Autodesk Fusion 360 part; units mm, degrees
(part 2 of 2)
sketch "Sketch7" plane through (-20, 0, 0) normal (-1, 0, 0) x (0, -1, 0) in component "ball"
  line L0 (15.0084, 21.0981) -> (-47.0084, 21.0981)
  line L1 (-45.8452, -1.5) -> (13.8452, -1.5)
  line L2 (-16, 21.0981) -> (-16, -1.5)
  spline S0 degree 5 poles (-16, 14) (-16.0768, 14.2889) (-16.2492, 14.8416) (-16.5647, 15.5947) (-17.0996, 16.4467) (-17.9572, 17.2552) (-18.9957, 17.8051) (-20.1949, 18.0972) (-21.5164, 18.1376) (-22.901, 17.9403) (-24.2811, 17.528) (-25.5916, 16.9332) (-26.7815, 16.2001) (-27.8246, 15.386) (-28.7338, 14.5642) (-29.5527, 13.8181) (-30.3405, 13.2309) (-31.1602, 12.878) (-32.064, 12.8165) (-33.0834, 13.0788) (-34.2362, 13.6807) (-35.2709, 14.4373) (-36.1107, 15.159) (-36.6989, 15.7083) (-37, 16) knots 0 0 0 0 0 0 0.05 0.1 0.15 0.2 0.25 0.3 0.35 0.4 0.45 0.5 0.55 0.6 0.65 0.7 0.75 0.8 0.85 0.9 0.95 1 1 1 1 1 1
  spline S1 degree 5 poles (-37, 16) (-37.054, 15.8762) (-37.1353, 15.6211) (-37.1776, 15.2158) (-37.0738, 14.6298) (-36.6785, 13.8269) (-36.0288, 12.9719) (-35.1528, 12.1033) (-34.1019, 11.2871) (-32.9409, 10.6016) (-31.738, 10.1239) (-30.5551, 9.9157) (-29.4385, 10.0096) (-28.4073, 10.3907) (-27.452, 10.9969) (-26.546, 11.7391) (-25.6526, 12.5164) (-24.7335, 13.2309) (-23.7575, 13.8057) (-22.7059, 14.1942) (-21.5684, 14.3708) (-20.5863, 14.3343) (-19.809, 14.2062) (-19.2727, 14.0762) (-19, 14) knots 0 0 0 0 0 0 0.05 0.1 0.15 0.2 0.25 0.3 0.35 0.4 0.45 0.5 0.55 0.6 0.65 0.7 0.75 0.8 0.85 0.9 0.95 1 1 1 1 1 1
  spline S2 degree 5 poles (-19, 14) (-19.1593, 13.9082) (-19.4654, 13.7188) (-19.8868, 13.4181) (-20.3668, 12.9863) (-20.8123, 12.4099) (-21.1083, 11.8121) (-21.3181, 11.2) (-21.5714, 10.5707) (-22.0076, 9.9217) (-22.7367, 9.2586) (-23.784, 8.6057) (-25.1061, 8.0019) (-26.6184, 7.4936) (-28.2175, 7.1291) (-29.8055, 6.952) (-31.3123, 6.9952) (-32.7222, 7.2735) (-34.063, 7.7868) (-35.3897, 8.5261) (-36.7709, 9.477) (-37.9734, 10.3947) (-38.9536, 11.1658) (-39.6449, 11.7159) (-40, 12) knots 0 0 0 0 0 0 0.05 0.1 0.15 0.2 0.25 0.3 0.35 0.4 0.45 0.5 0.55 0.6 0.65 0.7 0.75 0.8 0.85 0.9 0.95 1 1 1 1 1 1
  spline S3 degree 5 poles (-40, 12) (-39.9687, 11.8016) (-39.8965, 11.412) (-39.7599, 10.8497) (-39.5206, 10.1438) (-39.1227, 9.3355) (-38.6179, 8.6011) (-37.9915, 7.9389) (-37.2204, 7.3449) (-36.2794, 6.8136) (-35.1484, 6.3404) (-33.8195, 5.9223) (-32.3053, 5.5605) (-30.6447, 5.2605) (-28.8942, 5.0317) (-27.1214, 4.8852) (-25.3974, 4.8334) (-23.7904, 4.8877) (-22.359, 5.058) (-21.1435, 5.3502) (-20.1642, 5.7665) (-19.5763, 6.1986) (-19.2455, 6.5779) (-19.0737, 6.8552) (-19, 7) knots 0 0 0 0 0 0 0.05 0.1 0.15 0.2 0.25 0.3 0.35 0.4 0.45 0.5 0.55 0.6 0.65 0.7 0.75 0.8 0.85 0.9 0.95 1 1 1 1 1 1
  spline S4 degree 5 poles (-19, 7) (-19.0395, 6.762) (-19.1421, 6.3033) (-19.3671, 5.6668) (-19.795, 4.9205) (-20.4658, 4.1516) (-21.1809, 3.5372) (-21.8621, 3.0651) (-22.4694, 2.7196) (-23.0364, 2.481) (-23.646, 2.3283) (-24.3868, 2.2429) (-25.3204, 2.2114) (-26.4321, 2.2305) (-27.6344, 2.3056) (-28.8063, 2.4472) (-29.6176, 2.6233) (-30.1094, 2.7955) (-30.3795, 2.9288) (-30.5, 3) knots 0 0 0 0 0 0 0.066667 0.133333 0.2 0.266667 0.333333 0.4 0.466667 0.533333 0.6 0.666667 0.733333 0.8 0.866667 0.933333 1 1 1 1 1 1
  spline S5 degree 5 poles (-30.5, 3) (-30.428, 2.8413) (-30.2657, 2.5426) (-29.9676, 2.1509) (-29.4599, 1.7355) (-28.6407, 1.3622) (-27.6411, 1.096) (-26.4758, 0.9019) (-25.1766, 0.7599) (-23.7933, 0.6686) (-22.3845, 0.6374) (-21.0126, 0.6824) (-19.7366, 0.8207) (-18.6066, 1.0648) (-17.6554, 1.4167) (-16.8959, 1.8647) (-16.443, 2.287) (-16.1886, 2.633) (-16.0566, 2.8756) (-16, 3) knots 0 0 0 0 0 0 0.066667 0.133333 0.2 0.266667 0.333333 0.4 0.466667 0.533333 0.6 0.666667 0.733333 0.8 0.866667 0.933333 1 1 1 1 1 1
  spline S6 degree 5 poles (-16, 14) (-15.9232, 14.2889) (-15.7508, 14.8416) (-15.4353, 15.5947) (-14.9004, 16.4467) (-14.0428, 17.2552) (-13.0043, 17.8051) (-11.8051, 18.0972) (-10.4836, 18.1376) (-9.099, 17.9403) (-7.7189, 17.528) (-6.4084, 16.9332) (-5.2185, 16.2001) (-4.1754, 15.386) (-3.2662, 14.5642) (-2.4473, 13.8181) (-1.6595, 13.2309) (-0.8398, 12.878) (0.064, 12.8165) (1.0834, 13.0788) (2.2362, 13.6807) (3.2709, 14.4373) (4.1107, 15.159) (4.6989, 15.7083) (5, 16) knots 0 0 0 0 0 0 0.05 0.1 0.15 0.2 0.25 0.3 0.35 0.4 0.45 0.5 0.55 0.6 0.65 0.7 0.75 0.8 0.85 0.9 0.95 1 1 1 1 1 1
  line L3 (-15.2956, 11.3482) -> (-16.7044, 16.6518)
  line L4 (-34.3707, 13.4529) -> (-39.6293, 18.5471)
  line L5 (-16.7044, 11.3482) -> (-15.2956, 16.6518)
  line L6 (2.3707, 13.4529) -> (7.6293, 18.5471)
  spline S7 degree 5 poles (5, 16) (5.054, 15.8762) (5.1353, 15.6211) (5.1776, 15.2158) (5.0738, 14.6298) (4.6785, 13.8269) (4.0288, 12.9719) (3.1528, 12.1033) (2.1019, 11.2871) (0.9409, 10.6016) (-0.262, 10.1239) (-1.4449, 9.9157) (-2.5615, 10.0096) (-3.5927, 10.3907) (-4.548, 10.9969) (-5.454, 11.7391) (-6.3474, 12.5164) (-7.2665, 13.2309) (-8.2425, 13.8057) (-9.2941, 14.1942) (-10.4316, 14.3708) (-11.4137, 14.3343) (-12.191, 14.2062) (-12.7273, 14.0762) (-13, 14) knots 0 0 0 0 0 0 0.05 0.1 0.15 0.2 0.25 0.3 0.35 0.4 0.45 0.5 0.55 0.6 0.65 0.7 0.75 0.8 0.85 0.9 0.95 1 1 1 1 1 1
  line L7 (-36.4062, 17.3615) -> (-37.5938, 14.6385)
  line L8 (-21.2463, 14.6274) -> (-16.7537, 13.3726)
  line L9 (4.4062, 17.3615) -> (5.5938, 14.6385)
  line L10 (-10.7537, 14.6274) -> (-15.2463, 13.3726)
  spline S8 degree 5 poles (8, 12) (7.9687, 11.8016) (7.8965, 11.412) (7.7599, 10.8497) (7.5206, 10.1438) (7.1227, 9.3355) (6.6179, 8.6011) (5.9915, 7.9389) (5.2204, 7.3449) (4.2794, 6.8136) (3.1484, 6.3404) (1.8195, 5.9223) (0.3053, 5.5605) (-1.3553, 5.2605) (-3.1058, 5.0317) (-4.8786, 4.8852) (-6.6026, 4.8334) (-8.2096, 4.8877) (-9.641, 5.058) (-10.8565, 5.3502) (-11.8358, 5.7665) (-12.4237, 6.1986) (-12.7545, 6.5779) (-12.9263, 6.8552) (-13, 7) knots 0 0 0 0 0 0 0.05 0.1 0.15 0.2 0.25 0.3 0.35 0.4 0.45 0.5 0.55 0.6 0.65 0.7 0.75 0.8 0.85 0.9 0.95 1 1 1 1 1 1
  line L11 (-40.4106, 14.601) -> (-39.5894, 9.399)
  line L12 (-19.8094, 5.4101) -> (-18.1906, 8.5899)
  line L13 (8.4106, 14.601) -> (7.5894, 9.399)
  line L14 (-12.1906, 5.4101) -> (-13.8094, 8.5899)
  spline S9 degree 5 poles (-13, 7) (-12.9605, 6.762) (-12.8579, 6.3033) (-12.6329, 5.6668) (-12.205, 4.9205) (-11.5342, 4.1516) (-10.8191, 3.5372) (-10.1379, 3.0651) (-9.5306, 2.7196) (-8.9636, 2.481) (-8.354, 2.3283) (-7.6132, 2.2429) (-6.6796, 2.2114) (-5.5679, 2.2305) (-4.3656, 2.3056) (-3.1937, 2.4472) (-2.3824, 2.6233) (-1.8906, 2.7955) (-1.6205, 2.9288) (-1.5, 3) knots 0 0 0 0 0 0 0.066667 0.133333 0.2 0.266667 0.333333 0.4 0.466667 0.533333 0.6 0.666667 0.733333 0.8 0.866667 0.933333 1 1 1 1 1 1
  line L15 (-18.7185, 8.6976) -> (-19.2815, 5.3024)
  line L16 (-29.6914, 2.5221) -> (-31.3086, 3.4779)
  line L17 (-13.2815, 8.6976) -> (-12.7185, 5.3024)
  line L18 (-2.3086, 2.5221) -> (-0.6914, 3.4779)
  spline S10 degree 5 poles (-1.5, 3) (-1.572, 2.8413) (-1.7343, 2.5426) (-2.0324, 2.1509) (-2.5401, 1.7355) (-3.3593, 1.3622) (-4.3589, 1.096) (-5.5242, 0.9019) (-6.8234, 0.7599) (-8.2067, 0.6686) (-9.6155, 0.6374) (-10.9874, 0.6824) (-12.2634, 0.8207) (-13.3934, 1.0648) (-14.3446, 1.4167) (-15.1041, 1.8647) (-15.5571, 2.287) (-15.8114, 2.633) (-15.9434, 2.8756) (-16, 3) knots 0 0 0 0 0 0 0.066667 0.133333 0.2 0.266667 0.333333 0.4 0.466667 0.533333 0.6 0.666667 0.733333 0.8 0.866667 0.933333 1 1 1 1 1 1
  line L19 (-31.0931, 4.3075) -> (-29.9069, 1.6925)
  line L20 (-16.5066, 1.8872) -> (-15.4934, 4.1128)
  line L21 (-0.9069, 4.3075) -> (-2.0931, 1.6925)
  line L22 (-15.4934, 1.8872) -> (-16.5066, 4.1128)
  spline S11 degree 5 poles (-13, 14) (-12.8407, 13.9082) (-12.5346, 13.7188) (-12.1132, 13.4181) (-11.6332, 12.9863) (-11.1877, 12.4099) (-10.8917, 11.8121) (-10.6819, 11.2) (-10.4286, 10.5707) (-9.9924, 9.9217) (-9.2633, 9.2586) (-8.216, 8.6057) (-6.8939, 8.0019) (-5.3816, 7.4936) (-3.7825, 7.1291) (-2.1945, 6.952) (-0.6877, 6.9952) (0.7222, 7.2735) (2.063, 7.7868) (3.3897, 8.5261) (4.7709, 9.477) (5.9734, 10.3947) (6.9536, 11.1658) (7.6449, 11.7159) (8, 12) knots 0 0 0 0 0 0 0.05 0.1 0.15 0.2 0.25 0.3 0.35 0.4 0.45 0.5 0.55 0.6 0.65 0.7 0.75 0.8 0.85 0.9 0.95 1 1 1 1 1 1
  line L23 (-16.6348, 15.3636) -> (-21.3652, 12.6364)
  line L24 (-37.5, 10) -> (-42.5, 14)
  line L25 (-15.3652, 15.3636) -> (-10.6348, 12.6364)
  line L26 (5.5, 10) -> (10.5, 14)
  point P0 (-20, 18)
  point P1 (-27, 16)
  point P2 (-31, 13)
  point P3 (-36, 13)
  point P4 (-30, 10)
  point P5 (-25, 13)
  point P6 (-21, 12)
  point P7 (-22.1918, 9.799)
  point P8 (-30, 7)
  point P9 (-38.5308, 8.5504)
  point P10 (-34, 6)
  point P11 (-23, 5)
  point P12 (-22, 3)
  point P13 (-24.8082, 2.2362)
  point P14 (-27, 1)
  point P15 (-19, 1)
  point P16 (-12, 18)
  point P17 (-5, 16)
  point P18 (-1, 13)
  point P19 (4, 13)
  point P20 (-2, 10)
  point P21 (-7, 13)
  point P22 (6.5308, 8.5504)
  point P23 (2, 6)
  point P24 (-9, 5)
  point P25 (-10, 3)
  point P26 (-7.1918, 2.2362)
  point P27 (-5, 1)
  point P28 (-13, 1)
  point P29 (-11, 12)
  point P30 (-9.8082, 9.799)
  point P31 (-2, 7)
  constraint midpoint L0 L2.start
  constraint midpoint L1 L2.end
  constraint coincident L2 S0.start
  constraint coincident L2 S5.end
  constraint midpoint S0.start L3
  constraint midpoint S0.end L4
  constraint midpoint S0.end L7
  constraint midpoint S1.end L8
  constraint midpoint S2.end L11
  constraint midpoint S3.end L12
  constraint midpoint S3.end L15
  constraint midpoint S4.end L16
  constraint midpoint S4.end L19
  constraint midpoint S5.end L20
  constraint midpoint S1.end L23
  constraint midpoint S2.end L24
  constraint symmetric L2 S0.start S6.start
  constraint symmetric L2 P0 P16
  constraint symmetric L2 P1 P17
  constraint symmetric L2 P2 P18
  constraint symmetric L2 S0.end S6.end
  constraint symmetric L2 P3 P19
  constraint symmetric L2 P4 P20
  constraint symmetric L2 P5 P21
  constraint symmetric L2 S1.end S7.end
  constraint symmetric L2 P6 P29
  constraint symmetric L2 P7 P30
  constraint symmetric L2 P8 P31
  constraint symmetric L2 S2.end S8.start
  constraint symmetric L2 P9 P22
  constraint symmetric L2 P10 P23
  constraint symmetric L2 P11 P24
  constraint symmetric L2 S3.end S8.end
  constraint symmetric L2 P12 P25
  constraint symmetric L2 P13 P26
  constraint symmetric L2 S4.end S9.end
  constraint symmetric L2 P14 P27
  constraint symmetric L2 P15 P28
  constraint symmetric L2 S5.end S10.end
  constraint symmetric L2 L3.start L5.start
  constraint symmetric L2 L3.end L5.end
  constraint symmetric L2 L4.start L6.start
  constraint symmetric L2 L4.end L6.end
  constraint symmetric L2 L7.start L9.start
  constraint symmetric L2 L7.end L9.end
  constraint symmetric L2 L8.start L10.start
  constraint symmetric L2 L8.end L10.end
  constraint symmetric L2 L11.start L13.start
  constraint symmetric L2 L11.end L13.end
  constraint symmetric L2 L12.start L14.start
  constraint symmetric L2 L12.end L14.end
  constraint symmetric L2 L15.start L17.start
  constraint symmetric L2 L15.end L17.end
  constraint symmetric L2 L16.start L18.start
  constraint symmetric L2 L16.end L18.end
  constraint symmetric L2 L19.start L21.start
  constraint symmetric L2 L19.end L21.end
  constraint symmetric L2 L20.start L22.start
  constraint symmetric L2 L20.end L22.end
  constraint symmetric L2 L23.start L25.start
  constraint symmetric L2 L23.end L25.end
  constraint symmetric L2 L24.start L26.start
  constraint symmetric L2 L24.end L26.end
extrude "Extrude5'" cut sketch "Sketch7" against normal blind 25 bodies 2 in component "ball"
sketch "Sketch8" plane through (0, 0, 21.0981) normal (0, 0, 1) x (-1, 0, 0) in component "ball"
  circle A0 centre (-14.9383, -16) radius 31.0084
  circle A1 centre (-14.9383, -16) radius 29.4325
pattern_circular "C-Pattern1" count 3 over 360 about axis through (14.9566, 15.9909, -4.2) along (0, 0, 1) of "Extrude5'" in component "ball"
sketch "Sketch1 (4)" plane through (0, 0, -1.5) normal (0, 0, 1) x (-1, 0, 0) in component "extension"
  circle A0 centre (-42.0837, -16) radius 1
  circle A1 centre (12.2071, -16) radius 1
  circle A2 centre (-14.9383, -16) radius 29.8452
  arc A3 (13.1923, -13.9627) -> (-43.0689, -13.9627) centre (-14.9383, -16) ccw
  arc A4 (13.1923, -13.9627) -> (13.1923, -18.0373) centre (12.2071, -16) ccw
  arc A5 (-43.0689, -18.0373) -> (13.1923, -18.0373) centre (-14.9383, -16) ccw
  arc A6 (-43.0689, -18.0373) -> (-43.0689, -13.9627) centre (-42.0837, -16) ccw
  circle A7 centre (-14.9383, -16) radius 28.2043
  constraint concentric A2 A7
extrude "Extrude1'''" add sketch "Sketch1 (4)" along normal blind 10 separate body contours A2 makes body 6 in component "extension"
sketch "Sketch1 (5)" plane through (0, 16, 0) normal (0, 1, 0) x (1, 0, 0) in component "cap"
  spline S0 degree 3 poles (33.6875, -14) (34.5835, -14.3099) (35.3264, -14.3805) (36.6237, -14.1932) (37.1646, -13.937) (38.2798, -13.1441) (38.8055, -12.5318) (39.8448, -11.2941) (40.3568, -10.6687) (41.2779, -10.0864) (41.6509, -9.9614) (42.4833, -10.0177) (42.8832, -10.2011) (43.8376, -10.8937) (44.3591, -11.5742) (45.044, -12.8784) (45.2745, -13.5433) (45.4405, -14.5288) (45.458, -14.8297) (45.4481, -15.252) (45.4361, -15.408) (45.3915, -15.7167) (45.3607, -15.8616) (45.3214, -16) knots 0 0 0 0 0.347757 0.347757 0.693471 0.693471 1.163851 1.163851 1.680094 1.680094 1.993149 1.993149 2.311494 2.311494 2.845247 2.845247 3.301198 3.301198 3.550564 3.550564 3.691626 3.691626 3.827769 3.827769 3.827769 3.827769
  spline S1 degree 3 poles (45.3214, -16) (44.851, -14.667) (44.1735, -13.5705) (43.2036, -12.9208) (42.9372, -12.8567) (42.4624, -12.918) (42.2425, -13.0291) (41.7466, -13.4391) (41.4809, -13.7576) (40.4149, -15.1135) (39.2859, -16.6739) (36.5419, -17.9412) (35.6492, -18.1288) (34.2729, -18.0535) (33.7142, -17.9103) (32.7878, -17.3582) (32.4253, -17.0116) (31.8904, -16.2307) (31.7027, -15.8497) (31.3799, -14.9849) (31.2544, -14.4968) (31.1604, -14) knots 0 0 0 0 0.719439 0.719439 1.023307 1.023307 1.302416 1.302416 1.632983 1.632983 2.500728 2.500728 2.903769 2.903769 3.181925 3.181925 3.412664 3.412664 3.589293 3.589293 3.786428 3.786428 3.786428 3.786428
  spline S2 degree 3 poles (31.1604, -14) (30.9471, -14.7883) (30.625, -15.5542) (29.7972, -16.692) (29.3741, -17.0939) (28.3843, -17.7045) (27.849, -17.8961) (26.5454, -18.1356) (25.7656, -18.1111) (24.0487, -17.8187) (22.9402, -17.4516) (20.3642, -15.9895) (19.3561, -15.0245) (17.8649, -13.7598) (17.3075, -13.3425) (16.2925, -12.952) (15.8704, -12.8696) (14.94, -12.8938) (14.4385, -12.9877) (12.4362, -13.6838) (10.7904, -14.732) (8.9738, -16) knots 0 0 0 0 0.24545 0.24545 0.428593 0.428593 0.609942 0.609942 0.853396 0.853396 1.165598 1.165598 1.546937 1.546937 1.815146 1.815146 1.984101 1.984101 2.141432 2.141432 2.523706 2.523706 2.523706 2.523706
  spline S3 degree 3 poles (8.9738, -16) (8.9007, -15.8447) (8.8599, -15.682) (8.8432, -15.3308) (8.8718, -15.1525) (9.0066, -14.7139) (9.1484, -14.4577) (9.6196, -13.7713) (10.0734, -13.3075) (11.636, -11.9778) (13.104, -11.0415) (15.5333, -10.1392) (16.3608, -9.9836) (17.8575, -9.9873) (18.5032, -10.1416) (19.7788, -10.6838) (20.3858, -11.1044) (22.047, -12.4086) (23.0454, -13.384) (24.9981, -14.1786) (25.6423, -14.3085) (27.0539, -14.3401) (27.7918, -14.2124) (28.4941, -14) knots 0 0 0 0 0.051555 0.051555 0.106239 0.106239 0.191133 0.191133 0.360256 0.360256 0.704004 0.704004 0.918049 0.918049 1.127365 1.127365 1.370744 1.370744 1.820653 1.820653 2.036783 2.036783 2.278014 2.278014 2.278014 2.278014
  spline S4 degree 3 poles (28.4941, -14) (27.9198, -13.6274) (27.4521, -13.2065) (26.7871, -12.2856) (26.6289, -11.8776) (26.303, -10.9788) (26.134, -10.4635) (25.2167, -9.4348) (24.6854, -9.0762) (23.2362, -8.2376) (21.914, -7.7335) (19.1163, -7.0897) (17.2952, -6.8332) (13.104, -7.457) (11.3307, -8.4283) (8.376, -10.1195) (6.8875, -11.0228) (5.1481, -12) knots 0 0 0 0 0.223978 0.223978 0.425769 0.425769 0.683334 0.683334 0.903688 0.903688 1.384004 1.384004 1.830468 1.830468 2.346813 2.346813 2.720795 2.720795 2.720795 2.720795
  spline S5 degree 3 poles (5.1481, -12) (5.3651, -11.0862) (5.7294, -10.2289) (6.7885, -8.7676) (7.415, -8.205) (9.1019, -7.1287) (10.2386, -6.6768) (13.1879, -5.8121) (15.2978, -5.4029) (19.985, -4.8617) (22.0614, -4.7929) (24.8762, -5.0159) (25.9078, -5.2169) (27.0885, -5.7313) (27.4377, -5.9311) (28.0073, -6.4172) (28.2321, -6.6848) (28.3999, -7) knots 0 0 0 0 0.282973 0.282973 0.544611 0.544611 0.885334 0.885334 1.333576 1.333576 1.784582 1.784582 2.107176 2.107176 2.248199 2.248199 2.372209 2.372209 2.372209 2.372209
  spline S6 degree 3 poles (28.3999, -7) (28.2648, -6.3839) (28.0248, -5.7738) (27.2943, -4.6982) (26.8687, -4.2289) (25.9263, -3.4658) (25.5162, -3.1871) (24.3735, -2.5423) (23.792, -2.375) (22.1991, -2.1906) (20.9178, -2.2051) (19.0586, -2.3449) (18.3864, -2.419) (17.1043, -2.6679) (16.6547, -2.8222) (16.3428, -3) knots 0 0 0 0 0.189439 0.189439 0.338683 0.338683 0.43499 0.43499 0.611233 0.611233 0.834883 0.834883 0.9507 0.9507 1.077044 1.077044 1.077044 1.077044
  spline S7 degree 3 poles (16.3428, -3) (16.4515, -2.6984) (16.6108, -2.4295) (17.051, -1.962) (17.314, -1.7812) (17.9805, -1.4415) (18.4759, -1.2706) (20.4608, -0.8487) (22.4394, -0.6505) (25.8671, -0.6605) (27.3044, -0.8009) (28.9519, -1.4217) (29.4224, -1.6667) (30.0045, -2.1413) (30.1671, -2.2991) (30.4481, -2.6365) (30.5672, -2.8119) (30.6663, -3) knots 0 0 0 0 0.099523 0.099523 0.198309 0.198309 0.329298 0.329298 0.572591 0.572591 0.764033 0.764033 0.842721 0.842721 0.87626 0.87626 0.907407 0.907407 0.907407 0.907407
  spline S8 degree 3 poles (30.6663, -3) (30.7458, -2.6956) (30.8801, -2.4264) (31.2887, -1.8693) (31.5915, -1.6184) (32.4808, -1.0857) (33.1408, -0.9004) (35.0678, -0.5764) (36.6328, -0.6289) (38.7398, -0.9438) (39.5092, -1.12) (40.3992, -1.6121) (40.6501, -1.8101) (40.9801, -2.1866) (41.0833, -2.3273) (41.2776, -2.6453) (41.3647, -2.8178) (41.4421, -3) knots 0 0 0 0 0.103254 0.103254 0.245243 0.245243 0.492345 0.492345 1.006021 1.006021 1.302991 1.302991 1.4497 1.4497 1.524204 1.524204 1.600684 1.600684 1.600684 1.600684
  spline S9 degree 3 poles (41.4421, -3) (41.3064, -2.8844) (41.122, -2.7638) (40.3496, -2.4439) (39.668, -2.3157) (38.2978, -2.2122) (37.714, -2.2111) (36.6305, -2.3246) (36.2201, -2.4828) (35.558, -2.9993) (35.3403, -3.2054) (34.8188, -3.767) (34.4502, -4.2363) (34.0035, -5.1404) (33.8784, -5.4666) (33.6827, -6.1967) (33.6212, -6.5886) (33.5933, -7) knots 0 0 0 0 0.071077 0.071077 0.202116 0.202116 0.301066 0.301066 0.433215 0.433215 0.497193 0.497193 0.601672 0.601672 0.654922 0.654922 0.712197 0.712197 0.712197 0.712197
  spline S10 degree 3 poles (33.5933, -7) (33.6954, -6.7073) (33.8422, -6.4553) (34.2623, -5.9493) (34.5538, -5.731) (35.3777, -5.2712) (36.012, -5.0863) (37.9573, -4.7815) (39.5189, -4.829) (42.9628, -5.4691) (44.2979, -6.0911) (45.6177, -7.4892) (45.9305, -8.0788) (46.3114, -9.1921) (46.4296, -9.6814) (46.6082, -10.7829) (46.663, -11.3805) (46.685, -12) knots 0 0 0 0 0.099847 0.099847 0.232599 0.232599 0.463962 0.463962 0.892506 0.892506 1.441385 1.441385 1.761402 1.761402 1.968837 1.968837 2.183845 2.183845 2.183845 2.183845
  spline S11 degree 3 poles (46.685, -12) (46.1256, -10.5333) (45.2652, -9.1251) (43.7522, -7.5542) (43.0251, -7.1088) (41.1603, -6.9206) (40.1694, -7.2049) (38.4215, -7.9487) (37.5261, -8.4981) (36.3683, -9.5833) (36.0941, -10.005) (35.7431, -10.7177) (35.6431, -11.0736) (35.4034, -11.8712) (35.2559, -12.3177) (34.6195, -13.2447) (34.2072, -13.6444) (33.6875, -14) knots 0 0 0 0 0.936383 0.936383 1.666398 1.666398 2.412456 2.412456 3.226486 3.226486 3.826518 3.826518 4.477931 4.477931 5.331592 5.331592 6.127336 6.127336 6.127336 6.127336
  spline S12 degree 3 poles (28.4691, -14) (27.4442, -14.3098) (26.5497, -14.3804) (24.9605, -14.1933) (24.2802, -13.9372) (22.8431, -13.1447) (22.1327, -12.5327) (20.6229, -11.295) (19.815, -10.6691) (18.2636, -10.0866) (17.6166, -9.9616) (16.1106, -10.0174) (15.3545, -10.2005) (13.448, -10.8916) (12.2738, -11.5708) (10.4887, -12.8745) (9.7576, -13.5402) (9.091, -14.481) (8.9297, -14.7907) (8.8209, -15.2514) (8.8058, -15.4075) (8.8332, -15.7165) (8.873, -15.8614) (8.9382, -16) knots 0 0 0 0 0.347643 0.347643 0.693187 0.693187 1.163217 1.163217 1.679374 1.679374 1.992094 1.992094 2.310026 2.310026 2.842782 2.842782 3.298879 3.298879 3.515565 3.515565 3.623015 3.623015 3.726706 3.726706 3.726706 3.726706
  spline S13 degree 3 poles (8.9382, -16) (10.8501, -14.6665) (12.5794, -13.5699) (14.6815, -12.9207) (15.2141, -12.8567) (16.1229, -12.9181) (16.5239, -13.029) (17.3846, -13.4386) (17.8183, -13.7569) (19.4579, -15.1132) (21.0099, -16.6762) (24.4412, -17.9422) (25.5218, -18.1291) (27.1818, -18.053) (27.8542, -17.9095) (28.991, -17.357) (29.4454, -17.0103) (30.1357, -16.2292) (30.3855, -15.8485) (30.8247, -14.9841) (31.0023, -14.4964) (31.1366, -14) knots 0 0 0 0 0.7191 0.7191 1.022584 1.022584 1.301348 1.301348 1.631598 1.631598 2.499929 2.499929 2.902346 2.902346 3.180099 3.180099 3.410615 3.410615 3.586985 3.586985 3.783824 3.783824 3.783824 3.783824
  spline S14 degree 3 poles (31.1366, -14) (31.2859, -14.7883) (31.5143, -15.5542) (32.1445, -16.692) (32.4767, -17.094) (33.2759, -17.7046) (33.7172, -17.8961) (34.7972, -18.1356) (35.4463, -18.1111) (36.8558, -17.8185) (37.7534, -17.4512) (39.7475, -15.9882) (40.4738, -15.0229) (41.4595, -13.7588) (41.7987, -13.342) (42.3709, -12.9517) (42.5988, -12.8694) (43.074, -12.894) (43.3197, -12.9882) (44.2274, -13.6852) (44.861, -14.733) (45.3094, -16) knots 0 0 0 0 0.245461 0.245461 0.428639 0.428639 0.610036 0.610036 0.853579 0.853579 1.165847 1.165847 1.54722 1.54722 1.81505 1.81505 1.98398 1.98398 2.141333 2.141333 2.523101 2.523101 2.523101 2.523101
  spline S15 degree 3 poles (45.3094, -16) (45.3536, -15.8449) (45.3868, -15.6824) (45.4322, -15.3316) (45.4416, -15.1536) (45.4399, -14.7156) (45.4144, -14.4599) (45.3052, -13.7749) (45.1711, -13.3121) (44.6299, -11.9842) (44.0115, -11.0485) (42.8001, -10.1422) (42.3529, -9.9849) (41.5215, -9.986) (41.1498, -10.1363) (40.39, -10.6677) (40.0101, -11.0824) (38.9004, -12.3849) (38.1557, -13.3696) (36.6049, -14.1746) (36.0818, -14.307) (34.9102, -14.3412) (34.2823, -14.2134) (33.665, -14) knots 0 0 0 0 0.051503 0.051503 0.106111 0.106111 0.190848 0.190848 0.359591 0.359591 0.702822 0.702822 0.917286 0.917286 1.124895 1.124895 1.367315 1.367315 1.820839 1.820839 2.038753 2.038753 2.281958 2.281958 2.281958 2.281958
  spline S16 degree 3 poles (33.665, -14) (34.2099, -13.6274) (34.6391, -13.2065) (35.2399, -12.2856) (35.3786, -11.8775) (35.6517, -10.9788) (35.7848, -10.4635) (36.4778, -9.435) (36.8694, -9.0764) (37.9089, -8.2379) (38.8123, -7.734) (40.5613, -7.0899) (41.6275, -6.8331) (43.8442, -7.4589) (44.6739, -8.4373) (45.8085, -10.1242) (46.3028, -11.0253) (46.6763, -12) knots 0 0 0 0 0.223989 0.223989 0.425782 0.425782 0.683335 0.683335 0.903686 0.903686 1.383974 1.383974 1.830669 1.830669 2.349416 2.349416 2.72575 2.72575 2.72575 2.72575
  spline S17 degree 3 poles (46.6763, -12) (46.6436, -11.0864) (46.5403, -10.2295) (46.1893, -8.7685) (45.9675, -8.206) (45.3332, -7.1299) (44.8807, -6.6777) (43.5649, -5.8135) (42.5248, -5.405) (39.7485, -4.8619) (38.3066, -4.7925) (36.241, -5.0162) (35.4436, -5.2172) (34.5355, -5.7315) (34.2675, -5.9313) (33.8425, -6.4173) (33.6808, -6.6849) (33.5708, -7) knots 0 0 0 0 0.282943 0.282943 0.544668 0.544668 0.885418 0.885418 1.332124 1.332124 1.784181 1.784181 2.106506 2.106506 2.247435 2.247435 2.371367 2.371367 2.371367 2.371367
  spline S18 degree 3 poles (33.5708, -7) (33.6126, -6.384) (33.7327, -5.774) (34.1741, -4.6993) (34.4466, -4.2299) (35.0618, -3.4661) (35.3303, -3.1874) (36.0823, -2.5422) (36.4807, -2.3749) (37.6015, -2.1906) (38.4962, -2.2051) (39.7085, -2.3449) (40.1335, -2.419) (40.9359, -2.6679) (41.2167, -2.8223) (41.4255, -3) knots 0 0 0 0 0.189406 0.189406 0.338408 0.338408 0.434439 0.434439 0.610281 0.610281 0.833323 0.833323 0.948795 0.948795 1.074788 1.074788 1.074788 1.074788
  spline S19 degree 3 poles (41.4255, -3) (41.2974, -2.6985) (41.1453, -2.4297) (40.7832, -1.9624) (40.5875, -1.7815) (40.1125, -1.4418) (39.7759, -1.271) (38.4231, -0.8484) (37.0319, -0.6498) (34.3644, -0.661) (33.1718, -0.8018) (31.8512, -1.4228) (31.4814, -1.6677) (31.0575, -2.1419) (30.944, -2.2997) (30.7619, -2.6368) (30.6917, -2.812) (30.6426, -3) knots 0 0 0 0 0.099483 0.099483 0.198242 0.198242 0.329249 0.329249 0.573183 0.573183 0.76449 0.76449 0.843109 0.843109 0.876624 0.876624 0.907752 0.907752 0.907752 0.907752
  spline S20 degree 3 poles (30.6426, -3) (30.4821, -2.6956) (30.2704, -2.4265) (29.6871, -1.8695) (29.292, -1.6186) (28.1656, -1.0859) (27.3631, -0.9007) (24.9865, -0.5765) (22.9838, -0.6287) (20.0091, -0.9433) (18.8546, -1.1195) (17.5672, -1.6116) (17.2177, -1.8097) (16.7988, -2.1863) (16.6757, -2.327) (16.4627, -2.6451) (16.3776, -2.8177) (16.3119, -3) knots 0 0 0 0 0.103229 0.103229 0.245156 0.245156 0.492116 0.492116 1.005373 1.005373 1.302444 1.302444 1.44921 1.44921 1.523743 1.523743 1.600256 1.600256 1.600256 1.600256
  spline S21 degree 3 poles (16.3119, -3) (16.515, -2.8843) (16.8039, -2.7637) (18.0377, -2.4439) (19.1347, -2.3158) (21.1989, -2.2122) (22.0385, -2.211) (23.5808, -2.3246) (24.1717, -2.4827) (25.1746, -2.9988) (25.5076, -3.205) (26.305, -3.7664) (26.8674, -4.2358) (27.5849, -5.1401) (27.7944, -5.4664) (28.151, -6.1966) (28.2846, -6.5885) (28.3749, -7) knots 0 0 0 0 0.071123 0.071123 0.202326 0.202326 0.301499 0.301499 0.433869 0.433869 0.498001 0.498001 0.602731 0.602731 0.656106 0.656106 0.71352 0.71352 0.71352 0.71352
  spline S22 degree 3 poles (28.3749, -7) (28.219, -6.7073) (28.0137, -6.4553) (27.4478, -5.9493) (27.0679, -5.7311) (25.9963, -5.2713) (25.1744, -5.0863) (22.5568, -4.7815) (20.343, -4.829) (14.4889, -5.4781) (11.4767, -6.121) (8.2709, -7.558) (7.4251, -8.1404) (6.3587, -9.269) (6.0194, -9.748) (5.4593, -10.8197) (5.2521, -11.3997) (5.1094, -12) knots 0 0 0 0 0.09984 0.09984 0.232561 0.232561 0.463842 0.463842 0.892231 0.892231 1.454718 1.454718 1.754316 1.754316 1.939512 1.939512 2.131773 2.131773 2.131773 2.131773
  spline S23 degree 3 poles (5.1094, -12) (7.7236, -10.5327) (9.9081, -9.1247) (13.2407, -7.5544) (14.6823, -7.1092) (18.1051, -6.9204) (19.7639, -7.2043) (22.4998, -7.9471) (23.7819, -8.497) (25.3697, -9.5829) (25.7271, -10.0047) (26.1852, -10.7174) (26.3117, -11.0734) (26.6002, -11.8713) (26.7683, -12.3177) (27.4718, -13.2447) (27.9208, -13.6444) (28.4691, -14) knots 0 0 0 0 0.935585 0.935585 1.664592 1.664592 2.409964 2.409964 3.225511 3.225511 3.826201 3.826201 4.478452 4.478452 5.333957 5.333957 6.13181 6.13181 6.13181 6.13181
  spline S24 degree 3 poles (-17.3155, -14) (-17.187, -14.3098) (-17.0357, -14.3804) (-16.7444, -14.1933) (-16.6053, -13.9372) (-16.2838, -13.1447) (-16.0993, -12.5326) (-15.6296, -11.295) (-15.3343, -10.6691) (-14.7049, -10.0866) (-14.431, -9.9616) (-13.7577, -10.0174) (-13.4016, -10.2005) (-12.4498, -10.8918) (-11.7974, -11.5711) (-10.6993, -12.8748) (-10.2001, -13.5404) (-9.6928, -14.4811) (-9.558, -14.7908) (-9.4386, -15.2514) (-9.4116, -15.4075) (-9.3944, -15.7165) (-9.4034, -15.8615) (-9.4291, -16) knots 0 0 0 0 0.347651 0.347651 0.693206 0.693206 1.16326 1.16326 1.679422 1.679422 1.992164 1.992164 2.310124 2.310124 2.842947 2.842947 3.299034 3.299034 3.515711 3.515711 3.623164 3.623164 3.726858 3.726858 3.726858 3.726858
  spline S25 degree 3 poles (-9.4291, -16) (-10.869, -14.6666) (-11.9194, -13.5699) (-13.0504, -12.9207) (-13.3166, -12.8567) (-13.7504, -12.9181) (-13.9314, -13.029) (-14.2959, -13.4386) (-14.4639, -13.7569) (-15.0361, -15.1132) (-15.4567, -16.676) (-16.14, -17.9421) (-16.328, -18.1291) (-16.6117, -18.053) (-16.7255, -17.9095) (-16.936, -17.3571) (-17.0279, -17.0104) (-17.1834, -16.2293) (-17.2456, -15.8486) (-17.3623, -14.9842) (-17.4144, -14.4964) (-17.4547, -14) knots 0 0 0 0 0.719123 0.719123 1.022632 1.022632 1.30142 1.30142 1.63169 1.63169 2.499983 2.499983 2.902442 2.902442 3.180221 3.180221 3.410752 3.410752 3.587139 3.587139 3.783998 3.783998 3.783998 3.783998
  spline S26 degree 3 poles (-17.4547, -14) (-17.3906, -14.7883) (-17.2967, -15.5542) (-17.0988, -16.692) (-17.0077, -17.094) (-16.8166, -17.7045) (-16.7222, -17.8961) (-16.4978, -18.1356) (-16.3665, -18.1111) (-16.0581, -17.8185) (-15.8464, -17.4513) (-15.2626, -15.9883) (-14.9802, -15.023) (-14.4744, -13.7589) (-14.2562, -13.3421) (-13.8132, -12.9518) (-13.6185, -12.8694) (-13.162, -12.8939) (-12.9056, -12.9881) (-11.8098, -13.6851) (-10.7973, -14.7329) (-9.4291, -16) knots 0 0 0 0 0.245461 0.245461 0.428636 0.428636 0.61003 0.61003 0.853567 0.853567 1.16583 1.16583 1.547201 1.547201 1.815056 1.815056 1.983988 1.983988 2.14134 2.14134 2.523141 2.523141 2.523141 2.523141
  spline S27 degree 3 poles (-9.4291, -16) (-9.4003, -15.8449) (-9.3926, -15.6823) (-9.4212, -15.3316) (-9.4591, -15.1535) (-9.5917, -14.7155) (-9.7076, -14.4597) (-10.0684, -13.7746) (-10.3868, -13.3118) (-11.405, -11.9838) (-12.2527, -11.048) (-13.4718, -10.142) (-13.8542, -9.9848) (-14.5152, -9.9861) (-14.7842, -10.1365) (-15.2928, -10.668) (-15.5178, -11.0828) (-16.0759, -12.3854) (-16.3326, -13.3698) (-16.742, -14.1747) (-16.8659, -14.3071) (-17.1131, -14.3412) (-17.227, -14.2134) (-17.3155, -14) knots 0 0 0 0 0.051507 0.051507 0.106119 0.106119 0.190867 0.190867 0.359636 0.359636 0.702902 0.702902 0.917338 0.917338 1.124926 1.124926 1.367342 1.367342 1.820765 1.820765 2.038629 2.038629 2.281779 2.281779 2.281779 2.281779
  spline S28 degree 3 poles (-17.3155, -14) (-17.2858, -13.6274) (-17.2471, -13.2065) (-17.1826, -12.2856) (-17.163, -11.8775) (-17.11, -10.9788) (-17.0741, -10.4635) (-16.8496, -9.435) (-16.7097, -9.0764) (-16.2998, -8.2379) (-15.881, -7.734) (-14.831, -7.0899) (-14.0742, -6.8331) (-12.0859, -7.4588) (-11.1362, -8.437) (-9.3227, -10.1238) (-8.3305, -11.0251) (-6.9671, -12) knots 0 0 0 0 0.223989 0.223989 0.425782 0.425782 0.683336 0.683336 0.903689 0.903689 1.38398 1.38398 1.830653 1.830653 2.3493 2.3493 2.725624 2.725624 2.725624 2.725624
  spline S29 degree 3 poles (-6.9671, -12) (-7.1516, -11.0864) (-7.4127, -10.2294) (-8.1212, -8.7685) (-8.5262, -8.2059) (-9.5789, -7.1298) (-10.2636, -6.6776) (-11.8965, -5.8134) (-12.9619, -5.4049) (-14.8772, -4.8619) (-15.5194, -4.7926) (-16.2735, -5.0162) (-16.5076, -5.2172) (-16.7802, -5.7315) (-16.8614, -5.9313) (-17.0061, -6.4173) (-17.0693, -6.6848) (-17.1272, -7) knots 0 0 0 0 0.282945 0.282945 0.544664 0.544664 0.885464 0.885464 1.332424 1.332424 1.784563 1.784563 2.107015 2.107015 2.247997 2.247997 2.371977 2.371977 2.371977 2.371977
  spline S30 degree 3 poles (-17.1272, -7) (-17.0337, -6.384) (-16.9139, -5.774) (-16.6249, -4.6984) (-16.472, -4.2292) (-16.1439, -3.4661) (-16.0022, -3.1873) (-15.6105, -2.5423) (-15.4269, -2.3749) (-14.954, -2.1906) (-14.5668, -2.2051) (-13.9189, -2.3449) (-13.6715, -2.419) (-13.1911, -2.6679) (-13.022, -2.8223) (-12.9189, -3) knots 0 0 0 0 0.189408 0.189408 0.33867 0.33867 0.435011 0.435011 0.611411 0.611411 0.835168 0.835168 0.951012 0.951012 1.07741 1.07741 1.07741 1.07741
  spline S31 degree 3 poles (-12.9189, -3) (-12.8995, -2.6985) (-12.9067, -2.4297) (-12.9848, -1.9624) (-13.0521, -1.7815) (-13.2436, -1.4418) (-13.4025, -1.271) (-14.037, -0.8484) (-14.6302, -0.6499) (-15.393, -0.661) (-15.6365, -0.8017) (-15.9622, -1.4227) (-16.0625, -1.6677) (-16.2201, -2.1419) (-16.2691, -2.2997) (-16.3678, -2.6368) (-16.4166, -2.812) (-16.4667, -3) knots 0 0 0 0 0.099485 0.099485 0.198246 0.198246 0.329252 0.329252 0.573143 0.573143 0.764459 0.764459 0.843083 0.843083 0.8766 0.8766 0.907729 0.907729 0.907729 0.907729
  spline S32 degree 3 poles (-16.4667, -3) (-16.3856, -2.6956) (-16.3083, -2.4265) (-16.1338, -1.8695) (-16.0415, -1.6186) (-15.8046, -1.0859) (-15.6621, -0.9007) (-15.2126, -0.5765) (-14.7749, -0.6288) (-13.9096, -0.9433) (-13.5258, -1.1195) (-13.1299, -1.6116) (-13.0317, -1.8097) (-12.9432, -2.1863) (-12.9235, -2.3271) (-12.905, -2.6451) (-12.9072, -2.8177) (-12.9189, -3) knots 0 0 0 0 0.10323 0.10323 0.245162 0.245162 0.492131 0.492131 1.005416 1.005416 1.30248 1.30248 1.449243 1.449243 1.523774 1.523774 1.600285 1.600285 1.600285 1.600285
  spline S33 degree 3 poles (-12.9189, -3) (-12.986, -2.8843) (-13.0903, -2.7637) (-13.5514, -2.4439) (-13.9664, -2.3158) (-14.6596, -2.2122) (-14.9147, -2.211) (-15.3725, -2.3246) (-15.5529, -2.4827) (-15.8934, -2.9989) (-16.0085, -3.205) (-16.2841, -3.7665) (-16.4775, -4.2358) (-16.7478, -5.1402) (-16.8321, -5.4664) (-16.9928, -6.1966) (-17.0648, -6.5885) (-17.1272, -7) knots 0 0 0 0 0.07112 0.07112 0.202312 0.202312 0.301471 0.301471 0.433826 0.433826 0.497948 0.497948 0.602659 0.602659 0.656026 0.656026 0.713429 0.713429 0.713429 0.713429
  spline S34 degree 3 poles (-17.1272, -7) (-17.0734, -6.7073) (-17.015, -6.4553) (-16.8695, -5.9493) (-16.7812, -5.7311) (-16.5339, -5.2713) (-16.3466, -5.0863) (-15.6754, -4.7815) (-15.0242, -4.829) (-12.6662, -5.4781) (-11.0163, -6.1209) (-9.0961, -7.5578) (-8.5567, -8.1402) (-7.8614, -9.2689) (-7.634, -9.7479) (-7.2433, -10.8197) (-7.0884, -11.3997) (-6.9671, -12) knots 0 0 0 0 0.09984 0.09984 0.232564 0.232564 0.46385 0.46385 0.892249 0.892249 1.454723 1.454723 1.754409 1.754409 1.939671 1.939671 2.131999 2.131999 2.131999 2.131999
  spline S35 degree 3 poles (-6.9671, -12) (-9.019, -10.5328) (-10.3418, -9.1247) (-12.1595, -7.5544) (-12.8737, -7.1091) (-14.4311, -6.9204) (-15.0989, -7.2043) (-16.0858, -7.9472) (-16.4705, -8.4971) (-16.8987, -9.583) (-16.9817, -10.0047) (-17.0885, -10.7175) (-17.1149, -11.0735) (-17.1635, -11.8713) (-17.184, -12.3177) (-17.2507, -13.2447) (-17.2872, -13.6444) (-17.3155, -14) knots 0 0 0 0 0.935639 0.935639 1.664713 1.664713 2.410131 2.410131 3.225575 3.225575 3.826221 3.826221 4.478416 4.478416 5.333797 5.333797 6.131509 6.131509 6.131509 6.131509
  line L0 (-16.0701, -21.0981) -> (45.9467, -21.0981)
  line L1 (44.7834, 1.5) -> (-14.9069, 1.5)
  line L2 (14.9383, -21.0981) -> (14.9383, -44)
  circle A0 centre (14.9383, -11.3653) radius 32.5
  circle A1 centre (14.9383, -11.3653) radius 31
  line L3 (-16.0701, -21.0981) -> (45.9467, -21.0981)
  constraint midpoint L0 L2.start
  constraint perpendicular L0 L2
revolve "Revolve1'" add sketch "Sketch1 (5)" angle 360 about axis through (14.9383, 16, 21.0981) along (0, 0, 1) separate body contours L0 L2 A0 A1 L3 picked at (43.7945, -23.8444) makes body 7 in component "cap"
sketch "Sketch2 (4)" plane through (-20, 0, 0) normal (-1, 0, 0) x (0, -1, 0) in component "cap"
  spline S0 degree 5 poles (-3, 22) (-3.0117, 22.0801) (-3.0541, 22.2598) (-3.1749, 22.5874) (-3.4504, 23.1408) (-3.986, 24.0149) (-4.7142, 25.0354) (-5.6368, 26.1301) (-6.753, 27.2066) (-8.0574, 28.1655) (-9.5362, 28.9152) (-11.1651, 29.3858) (-12.9055, 29.545) (-14.7088, 29.3971) (-16.5238, 28.9744) (-18.3035, 28.3312) (-20.0119, 27.5371) (-21.6305, 26.6707) (-23.1666, 25.8125) (-24.6535, 25.0397) (-26.134, 24.423) (-27.6494, 24.0232) (-29.2242, 23.8874) (-30.8554, 24.0463) (-32.495, 24.509) (-34.0529, 25.2637) (-35.4173, 26.2801) (-36.47, 27.512) (-37.1039, 28.8997) (-37.2395, 30.3725) (-36.8421, 31.8509) (-35.9204, 33.2509) (-34.5225, 34.4897) (-32.7336, 35.4891) (-30.6732, 36.1815) (-28.4929, 36.5138) (-26.3716, 36.4524) (-24.4933, 35.9887) (-23.028, 35.1439) (-22.1099, 33.9745) (-21.8193, 32.5768) (-22.1576, 31.0956) (-23.0398, 29.7174) (-24.3244, 28.631) (-25.8357, 27.9929) (-27.3885, 27.8932) (-28.8131, 28.3146) (-29.9747, 29.115) (-30.7684, 30.0886) (-31.1183, 31.0141) (-30.9752, 31.7075) (-30.4471, 32.0021) (-29.8152, 32.0632) (-29.2892, 32.0329) (-29, 32) knots 0 0 0 0 0 0 0.02 0.04 0.06 0.08 0.1 0.12 0.14 0.16 0.18 0.2 0.22 0.24 0.26 0.28 0.3 0.32 0.34 0.36 0.38 0.4 0.42 0.44 0.46 0.48 0.5 0.52 0.54 0.56 0.58 0.6 0.62 0.64 0.66 0.68 0.7 0.72 0.74 0.76 0.78 0.8 0.82 0.84 0.86 0.88 0.9 0.92 0.94 0.96 0.98 1 1 1 1 1 1
  spline S1 degree 5 poles (-29, 32) (-29.0202, 31.8673) (-29.0241, 31.6237) (-28.9201, 31.3235) (-28.5626, 31.0541) (-27.7872, 30.932) (-26.8047, 31.0144) (-25.8314, 31.2808) (-25.0998, 31.7006) (-24.8045, 32.2332) (-25.0226, 32.8264) (-25.7015, 33.4185) (-26.72, 33.9432) (-27.9297, 34.3332) (-29.2095, 34.5246) (-30.4678, 34.4637) (-31.6323, 34.1146) (-32.6445, 33.4682) (-33.4525, 32.5476) (-34.0027, 31.4203) (-34.2416, 30.1915) (-34.1265, 28.9823) (-33.6356, 27.9119) (-32.7758, 27.0799) (-31.596, 26.5435) (-30.1831, 26.3148) (-28.6432, 26.3733) (-27.0879, 26.6749) (-25.6175, 27.1617) (-24.3069, 27.7718) (-23.1868, 28.4495) (-22.2393, 29.1517) (-21.4158, 29.8448) (-20.6507, 30.505) (-19.8759, 31.1164) (-19.0355, 31.6708) (-18.0987, 32.1657) (-17.0535, 32.6015) (-15.9041, 32.9783) (-14.6667, 33.2928) (-13.3661, 33.5348) (-12.0318, 33.6847) (-10.6964, 33.7161) (-9.3931, 33.599) (-8.1544, 33.3023) (-7.0094, 32.7966) (-5.9823, 32.0575) (-5.0907, 31.0676) (-4.3467, 29.8147) (-3.7582, 28.2914) (-3.3298, 26.4935) (-3.1167, 24.8342) (-3.0299, 23.4655) (-3.0046, 22.4977) (-3, 22) knots 0 0 0 0 0 0 0.02 0.04 0.06 0.08 0.1 0.12 0.14 0.16 0.18 0.2 0.22 0.24 0.26 0.28 0.3 0.32 0.34 0.36 0.38 0.4 0.42 0.44 0.46 0.48 0.5 0.52 0.54 0.56 0.58 0.6 0.62 0.64 0.66 0.68 0.7 0.72 0.74 0.76 0.78 0.8 0.82 0.84 0.86 0.88 0.9 0.92 0.94 0.96 0.98 1 1 1 1 1 1
  spline S2 degree 5 poles (-20.2205, 38.2828) (-20.2657, 38.4037) (-20.3393, 38.6376) (-20.3992, 38.965) (-20.3778, 39.3547) (-20.1823, 39.762) (-19.8233, 40.0873) (-19.3141, 40.3273) (-18.6808, 40.4781) (-17.9584, 40.5368) (-17.186, 40.5038) (-16.4018, 40.385) (-15.639, 40.1939) (-14.9208, 39.9548) (-14.2569, 39.703) (-13.6477, 39.4795) (-13.0873, 39.3262) (-12.5667, 39.2816) (-12.077, 39.3764) (-11.612, 39.6283) (-11.168, 40.0462) (-10.8278, 40.5153) (-10.5807, 40.9428) (-10.4196, 41.2612) (-10.34, 41.4288) knots 0 0 0 0 0 0 0.05 0.1 0.15 0.2 0.25 0.3 0.35 0.4 0.45 0.5 0.55 0.6 0.65 0.7 0.75 0.8 0.85 0.9 0.95 1 1 1 1 1 1
  spline S3 degree 5 poles (-10.34, 41.4288) (-10.2547, 41.3278) (-10.1036, 41.1231) (-9.9347, 40.8089) (-9.8258, 40.3752) (-9.8835, 39.8107) (-10.1298, 39.2309) (-10.5514, 38.65) (-11.1203, 38.0934) (-11.7967, 37.5954) (-12.5353, 37.192) (-13.2913, 36.9151) (-14.0265, 36.7862) (-14.7152, 36.8096) (-15.3508, 36.9654) (-15.9416, 37.2159) (-16.5046, 37.5143) (-17.0609, 37.8125) (-17.63, 38.0691) (-18.2243, 38.2576) (-18.851, 38.3632) (-19.3807, 38.3763) (-19.7943, 38.3454) (-20.0772, 38.3067) (-20.2205, 38.2828) knots 0 0 0 0 0 0 0.05 0.1 0.15 0.2 0.25 0.3 0.35 0.4 0.45 0.5 0.55 0.6 0.65 0.7 0.75 0.8 0.85 0.9 0.95 1 1 1 1 1 1
  line L0 (-17.1142, 40.5669) -> (-14.6752, 39.9313)
  line L1 (-15.9565, 37.2686) -> (-18.2401, 38.369)
  point P0 (-4, 24)
  point P1 (-10, 29)
  point P2 (-21, 27)
  point P3 (-30, 24)
  point P4 (-37, 29)
  point P5 (-31, 36)
  point P6 (-22, 33)
  point P7 (-27, 28)
  point P8 (-31, 31)
  point P9 (-28, 31)
  point P10 (-25, 32)
  point P11 (-27, 34)
  point P12 (-33, 33)
  point P13 (-33.1849, 27.5508)
  point P14 (-24.8295, 27.5508)
  point P15 (-20, 31)
  point P16 (-14.7051, 33.2626)
  point P17 (-7.3118, 32.8863)
  point P18 (-19.7289, 40.1016)
  point P19 (-15.8947, 40.2491)
  point P20 (-12.6012, 39.3151)
  point P21 (-10.34, 38.971)
  point P22 (-14.0983, 36.8188)
  point P23 (-17.0983, 37.8188)
  constraint midpoint P19 L0
  constraint midpoint P23 L1
extrude "Extrude1''''" cut sketch "Sketch2 (4)" against normal blind 34 bodies 7 in component "cap"
pattern_circular "C-Pattern1'" count 3 over 360 about axis through (14.9566, 15.9909, -4.2) along (0, 0, 1) of "Extrude1''''" in component "cap"
sketch "Sketch1 (6)" plane through (0, 16, 0) normal (0, 1, 0) x (1, 0, 0) in component "hinge"
  circle A0 centre (14.9383, -11.3653) radius 32.5
  circle A1 centre (51.3601, -22.7392) radius 2.5
  line L0 (46.3422, -19.7347) -> (49.0843, -21.7044)
  line L1 (53.3007, -21.1631) -> (51.843, -19.3683)
  line L2 (51.843, -19.3683) -> (47.1106, -15.969)
  dimension "d80" = 5
  constraint coincident A0 L0.start
  constraint coincident A1 L0.end
  constraint coincident A1 L1.start
  constraint tangent A1 L1
  constraint coincident A0 L2.end
  constraint parallel L0 L2
  measures "d80" diameter of A1
extrude "Extrude1'''''" add sketch "Sketch1 (6)" along normal mid plane 12 separate body contours A0 A1 L0 L1 L2 | A1 makes body 8 in component "hinge"
sketch "Sketch2 (5)" plane through (0, 16, 0) normal (0, 1, 0) x (1, 0, 0) in component "hinge"
ref_plane "WorkPlane1" through (50.4966, 16, 20.9868) normal (0, -1, 0) x (-1, 0, 0) in component "hinge"
sketch "Sketch3 (3)" plane through (0, 16, 0) normal (0, -1, 0) x (-1, 0, 0) in component "hinge"
  arc A0 (-53.3007, -21.1631) -> (-49.0843, -21.7044) centre (-51.3601, -22.7392) ccw
  circle A1 centre (-51.3601, -22.7392) radius 2.5
  constraint concentric A0 A1
extrude "Extrude2'''" cut sketch "Sketch3 (3)" along normal mid plane 5 bodies 8 in component "hinge"
sketch "Sketch4 (3)" plane through (0, 16, 0) normal (0, -1, 0) x (-1, 0, 0) in component "hinge"
  arc A0 (-53.3007, -21.1631) -> (-49.0843, -21.7044) centre (-51.3601, -22.7392) ccw
  circle A1 centre (-51.3601, -22.7392) radius 1.75
  dimension "d85" = 3.5
  constraint concentric A0 A1
  measures "d85" diameter of A1
extrude "Extrude3''" cut sketch "Sketch4 (3)" along normal mid plane 10 bodies 8 in component "hinge"
sketch "Sketch5 (3)" plane through (0, 16, 0) normal (0, -1, 0) x (-1, 0, 0) in component "hinge"
  circle A0 centre (-14.9383, -11.3653) radius 32.5
  arc A1 (-53.3007, -21.1631) -> (-49.0843, -21.7044) centre (-51.3601, -22.7392) ccw
  circle A2 centre (-51.3601, -22.7392) radius 0.75
  line L0 (-51.6785, -23.4183) -> (-43.3935, -27.0673)
  line L1 (-51.1407, -22.022) -> (-45.4491, -22.5609)
  dimension "d88" = 1.5
  constraint concentric A1 A2
  constraint coincident A2 L0.start
  constraint coincident A0 L0.end
  constraint coincident A2 L1.start
  constraint coincident A0 L1.end
  measures "d88" diameter of A2
extrude "Extrude4''" add sketch "Sketch5 (3)" along normal mid plane 8 separate body contours A2 makes body 9 in component "hinge"
extrude "Extrude5''" add sketch "Sketch5 (3)" along normal mid plane 4 contours A0 A1 L0 L1 | A1 A2 L0 L1 bodies 9 in component "hinge"
combine "Combine1" operation cut target body 8 tool bodies 2 body 2 seen with x (1, 0, 0) y (0, 1, 0) z (0, 0, 1) at (0.7724, 0, 0.2357) keep tools in component "hinge"
combine "Combine2" operation cut target body 9 tool bodies 7 body 7 seen with x (1, 0, 0) y (0, 1, 0) z (0, 0, 1) at (0.7724, 0, 0.2357) keep tools in component "hinge"
copy_body "Body->Comp1'" bodies 9 removing the originals makes body 10 in component "hinge2"
component "base" placed x (1, 0, 0) y (0, 1, 0) z (0, 0, 1) at (0, 0, 0)
component "ball" placed x (1, 0, 0) y (0, 1, 0) z (0, 0, 1) at (0, 0, 0)
component "cap" placed x (1, 0, 0) y (0, 1, 0) z (0, 0, 1) at (0, 0, 0)
component "hinge" placed x (1, 0, 0) y (0, 1, 0) z (0, 0, 1) at (-0.7724, 0, -0.2357)
component "hinge2" placed x (1, 0, 0) y (0, 1, 0) z (0, 0, 1) at (-0.7724, 0, -0.2357)
component "bottom sphere" placed x (1, 0, 0) y (0, 1, 0) z (0, 0, 1) at (0, 0, 0) in component "ball"
component "extension" placed x (1, 0, 0) y (0, 1, 0) z (0, 0, 1) at (0, 0, 0) in component "bottom sphere"
